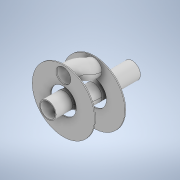
# Autodesk Inventor part: Combined_Intake_Exhaust_Manifold_2_0
Saved by Autodesk Inventor 2021 (Build 250183000, 183)
## iProperties
Created: 2021-04-23
Part Number: Combined_Intake_Exhaust_Manifold_2_0
Material: Generic
Document SubType Name: Modeling
Designer: lucia
Density: 1 g/cm^3
Appearance: Default
Author: lucia
Autodesk Inventor part; units mm, degrees
ref_plane "YZ Plane" through (0, 0, 0) normal (1, 0, 0) x (0, 1, 0)
ref_plane "XZ Plane" through (0, 0, 0) normal (0, 1, 0) x (-1, 0, 0)
sketch "Sketch1" plane through (0, 0, 0) normal (0, 0, 1) x (1, 0, 0)
  line L0 (0, 0) -> (0, -13.208)
  circle A0 centre (0, -13.208) radius 8.128
  circle A1 centre (0, -13.208) radius 12.7
  circle A2 centre (0, -13.208) radius 14.2875
  dimension "d0" = 13.208
  dimension "d1" = 16.256
  dimension "d2" = 25.4
  dimension "d3" = 28.575
  constraints: 3 centre point, 3 coincident, 2 end point, 1 vertical
  measures "d0" distance of L0.start L0.end
  measures "d1" diameter of A0
  measures "d2" diameter of A1
  measures "d3" diameter of A2
extrude "Extrusion1" add sketch "Sketch1" along normal blind 66.675 contours A2
sketch "Sketch2" plane through (0, 0, 0) normal (0, 0, 1) x (1, 0, 0)
  line L0 (0, 0) -> (0, -13.208)
  circle A0 centre (0, -13.208) radius 8.128
  circle A1 centre (0, -13.208) radius 12.7
  circle A2 centre (0, -13.208) radius 14.2875
  circle A3 centre (0, 18.542) radius 12.7
  circle A4 centre (0, 18.542) radius 14.2875
  dimension "d7" = 13.208
  dimension "d8" = 16.256
  dimension "d9" = 25.4
  dimension "d10" = 28.575
  dimension "d12" = 31.75
  dimension "d13" = 25.4
  dimension "d14" = 28.575
  constraints: 5 centre point, 4 coincident, 2 end point, 1 vertical
  measures "d7" distance of L0.start L0.end
  measures "d8" diameter of A0
  measures "d9" diameter of A1
  measures "d10" diameter of A2
  measures "d12" distance of L0.end A3.centre
  measures "d13" diameter of A3
  measures "d14" diameter of A4
sketch "Sketch3" plane through (0, 0, 0) normal (1, 0, 0) x (0, 1, 0)
  line L0 (1.0795, 66.675) -> (-27.4955, 66.675) projected
  line L1 (-13.208, 66.675) -> (-13.208, 98.425) construction
  line L2 (-13.208, 98.425) -> (0, 98.425) construction
  line L3 (0, 98.425) -> (0, 117.475) construction
  spline S0 degree 3 poles (-13.208, 66.675) (-13.208, 98.425) (0, 98.425) (0, 117.475) knots 1 1 1 1 2 2 2 2
  line L4 (24.892, 66.675) -> (24.892, 85.725) construction
  line L5 (24.892, 85.725) -> (38.1, 85.725) construction
  line L6 (38.1, 85.725) -> (38.1, 117.475) construction
  spline S1 degree 3 poles (24.892, 66.675) (24.892, 85.725) (38.1, 85.725) (38.1, 117.475) knots 1 1 1 1 2 2 2 2
  point P0 (0, 0)
  dimension "d15" = 13.208
  dimension "d16" = 31.75
  dimension "d17" = 19.05
  dimension "d28" = 13.208
  dimension "d31" = 31.75
  dimension "d32" = 19.05
  dimension "d34" = 38.1
  constraints: 4 vertical, 2 horizontal, 1 midpoint, 6 other
  measures "d15" distance of L1.end L2.end
  measures "d16" distance of L1.start L1.end
  measures "d17" distance of L2.end L3.end
  measures "d28" distance of L4.end L5.end
  measures "d31" distance of L5.end L6.end
  measures "d32" distance of L4.start L4.end
  measures "d34" distance of L3.end L6.end
ref_plane "Work Plane1" through (0, 0, 66.675) normal (0, 0, 1) x (1, 0, 0)
sketch "Sketch4" plane through (0, 0, 66.675) normal (0, 0, 1) x (1, 0, 0)
  line L0 (0, 0) -> (0, -13.208)
  circle A0 centre (0, -13.208) radius 8.128
  circle A1 centre (0, -13.208) radius 12.7
  circle A2 centre (0, -13.208) radius 14.2875
  circle A3 centre (0, 24.892) radius 12.7
  circle A4 centre (0, 24.892) radius 14.2875
  dimension "d19" = 13.208
  dimension "d20" = 16.256
  dimension "d21" = 25.4
  dimension "d22" = 28.575
  dimension "d23" = 38.1
  dimension "d24" = 25.4
  dimension "d25" = 28.575
  constraints: 5 centre point, 4 coincident, 2 end point, 1 vertical
  measures "d19" distance of L0.start L0.end
  measures "d20" diameter of A0
  measures "d21" diameter of A1
  measures "d22" diameter of A2
  measures "d23" distance of L0.end A3.centre
  measures "d24" diameter of A3
  measures "d25" diameter of A4
sweep "Sweep1" add profiles "Sketch4" path "Sketch3" path curves S0 contours A2
sweep "Sweep2" add profiles "Sketch4" path "Sketch3" path curves S1 contours A4
sketch "Sketch5" plane through (0, 0, 66.675) normal (0, 0, 1) x (1, 0, 0)
  line L0 (0, 0) -> (0, -13.208)
  circle A0 centre (0, -13.208) radius 8.128
  circle A1 centre (0, -13.208) radius 12.7
  circle A2 centre (0, -13.208) radius 14.2875
  circle A3 centre (0, 24.892) radius 12.7
  circle A4 centre (0, 24.892) radius 14.2875
  circle A5 centre (0, -13.208) radius 12.7 projected
  circle A6 centre (0, -13.208) radius 53.975
  circle A7 centre (0, -13.208) radius 22.225
  dimension "d39" = 13.208
  dimension "d40" = 16.256
  dimension "d41" = 25.4
  dimension "d42" = 28.575
  dimension "d43" = 38.1
  dimension "d44" = 25.4
  dimension "d45" = 28.575
  dimension "d47" = 107.95
  dimension "d56" = 44.45
  constraints: 7 centre point, 6 coincident, 2 end point, 1 vertical
  measures "d39" distance of L0.start L0.end
  measures "d40" diameter of A0
  measures "d41" diameter of A1
  measures "d42" diameter of A2
  measures "d43" distance of L0.end A3.centre
  measures "d44" diameter of A3
  measures "d45" diameter of A4
  measures "d47" diameter of A6
  measures "d56" diameter of A7
extrude "Extrusion2" add sketch "Sketch5" against normal blind 1.5875 contours A4 | A6
ref_plane "Work Plane2" through (0, 0, 117.475) normal (0, 0, 1) x (1, 0, 0)
sketch "Sketch6" plane through (0, 0, 117.475) normal (0, 0, 1) x (1, 0, 0)
  circle A0 centre (0, 0) radius 12.7
  circle A1 centre (0, 0) radius 14.2875
  dimension "d51" = 25.4
  dimension "d52" = 28.575
  constraints: 2 centre point, 2 coincident
  measures "d51" diameter of A0
  measures "d52" diameter of A1
extrude "Extrusion3" add sketch "Sketch6" along normal blind 28.575
sketch "Sketch7" plane through (0, 0, 117.475) normal (0, 0, 1) x (1, 0, 0)
  circle A0 centre (0, 0) radius 12.7
  circle A1 centre (0, 0) radius 14.2875
  circle A2 centre (0, 0) radius 22.225
  circle A3 centre (0, 0) radius 53.975
  circle A4 centre (0, 38.1) radius 12.7
  circle A5 centre (0, 38.1) radius 14.2875
  dimension "d57" = 25.4
  dimension "d58" = 28.575
  dimension "d59" = 38.1
  dimension "d60" = 28.575
  dimension "d61" = 25.4
  dimension "d62" = 44.45
  dimension "d63" = 107.95
  constraints: 6 centre point, 5 coincident
  measures "d57" diameter of A0
  measures "d58" diameter of A1
  measures "d59" distance of point (0, 0) A4.centre
  measures "d60" diameter of A5
  measures "d61" diameter of A4
  measures "d62" diameter of A2
  measures "d63" diameter of A3
extrude "Extrusion4" add sketch "Sketch7" along normal blind 1.5875 contours A3 | A5
equation "\"d0\" = 3.302 * d4"
equation "\"d1\" = 4.064 * d4"
equation "\"d2\" = 6.35 * d4"
equation "\"d7\" = 3.302 * d11"
equation "\"d8\" = 4.064 * d11"
equation "\"d9\" = 6.35 * d11"
equation "\"d15\" = 3.302 * scale"
equation "\"d16\" = first"
equation "\"d28\" = 3.302 * scale"
equation "\"d31\" = first"
equation "\"d19\" = 3.302 * d26"
equation "\"d20\" = 4.064 * d26"
equation "\"d21\" = 6.35 * d26"
equation "\"d39\" = 3.302 * d46"
equation "\"d40\" = 4.064 * d46"
equation "\"d41\" = 6.35 * d46"
equation "\"first\" = 31.75"
equation "\"d4\" = 4"
equation "\"d11\" = 4"
equation "\"scale\" = 4"
equation "\"d26\" = 4"
equation "\"d46\" = 4"
body "Solid1"
